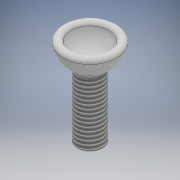
# Autodesk Inventor part: Component 28 (Rocker Arm Linkage)
Saved by Autodesk Inventor 2018 (Build 220112000, 112)
## iProperties
Created: 2023-03-30
Part Number: Component 28 (Rocker Arm Linkage)
Material: Generic
Document SubType Name: Modeling
Designer: Habib Mohamed
Density: 1 g/cm^3
Appearance: Default
Author: Habib Mohamed
Autodesk Inventor part; units mm, degrees
ref_plane "YZ Plane" through (0, 0, 0) normal (1, 0, 0) x (0, 1, 0)
ref_plane "XZ Plane" through (0, 0, 0) normal (0, 1, 0) x (-1, 0, 0)
ref_plane "XY Plane" through (0, 0, 0) normal (0, 0, 1) x (1, 0, 0)
sketch "Sketch1" plane through (0, 0, 0) normal (1, 0, 0) x (0, 1, 0)
  line L0 (0, 4.625) -> (0, -4.625)
  line L1 (0, -4.625) -> (1.625, -4.625)
  line L2 (1.625, -4.625) -> (1.625, 3.7361)
  arc A0 (1.8594, 4.1597) -> (3.5, 7.125) centre (0, 7.125) ccw
  arc A1 (0, 4.625) -> (2.5, 7.125) centre (0, 7.125) ccw
  line L3 (2.5, 7.125) -> (3.5, 7.125)
  arc A2 (1.8594, 4.1597) -> (1.625, 3.7361) centre (2.125, 3.7361) ccw
  point P0 (0, 0)
  point P1 (1.625, 4.0251)
  dimension "d0" = 11.75
  dimension "d1" = 1.625
  dimension "d2" = 2.5
  dimension "d3" = 3.5
  dimension "d4" = 0.5
  constraints: 8 end point, 7 point on circle, 3 centre point, 3 point on line, 2 midpoint, 2 perpendicular, 2 tangent, 1 coincident, 1 horizontal, 1 vertical
  measures "d0" distance between parallel lines of L1 L3
  measures "d1" distance of L0.end L1.end
  measures "d2" radius of A1
  measures "d3" radius of A0
  measures "d4" radius of A2
revolve "Revolution1" add sketch "Sketch1" angle 360 about axis through (0, 0, 4.625) along (0, 0, -1)
sketch "Sketch2" plane through (0, 0, -4.625) normal (0, 0, -1) x (-1, 0, 0)
  circle A0 centre (0, 0) radius 1.625 projected
  line L0 (0.5774, 1) -> (1.1547, 0)
  line L1 (1.1547, 0) -> (0.5774, -1)
  line L2 (0.5774, -1) -> (-0.5774, -1)
  line L3 (-0.5774, -1) -> (-1.1547, 0)
  line L4 (-1.1547, 0) -> (-0.5774, 1)
  line L5 (-0.5774, 1) -> (0.5774, 1)
  point P0 (0, 0)
  dimension "d6" = 2
  constraints: 12 end point, 1 coincident, 13 other
  measures "d6" distance between parallel lines of L2 L5
extrude "Extrusion1" cut sketch "Sketch2" against normal blind 1.5 contours L0 L1 L2 L3 L4 L5
fillet "Fillet1" radius 0.2 1 edges at (0, -1.625, -4.625)
fillet "Fillet2" radius 0.5 2 edges at (0, -3.5, 7.125) (0, -2.5, 7.125)
thread "Thread2" size "M4x0.5" class "6g" standard "ANSI Metric M Profile" length 8.161
body "Solid1"
